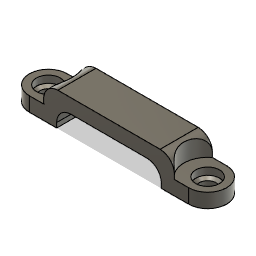
wireholder (Autodesk Fusion 360 design; units mm, degrees)
Autodesk Fusion 360 part; units mm, degrees
note: some values were not read from the file. Set by a fixed rule: which sketch regions a step uses.
sketch "Sketch1" plane through (0, 0, 0) normal (0, 1, 0) x (1, 0, 0)
  line L0 (0, 0) -> (33.5, 0)
  circle A0 centre (0, 0) radius 1.75
  circle A1 centre (33.5, 0) radius 1.75
  circle A2 centre (33.5, 0) radius 4
  circle A3 centre (0, 0) radius 4
  line L1 (0, 4) -> (33.5, 4)
  line L2 (33.5, -4) -> (0, -4)
  dimension "d1" = 33.5
  dimension "d2" = 3.5
  dimension "d3" = 3.5
  dimension "d4" = 8
  dimension "d5" = 8
  constraint coincident L0.start A0.centre
  constraint horizontal L0
  constraint coincident L0.end A1.centre
  constraint concentric A1 A2
  constraint coincident A3 L1.start
  constraint coincident A2 L1.end
  constraint tangent A2 L1
  constraint parallel L0 L1
  constraint coincident A2 L2.start
  constraint coincident A3 L2.end
  constraint tangent A3 L2
  constraint parallel L1 L2
  measures "d1" distance of L0.start L0.end
  measures "d2" diameter of A0
  measures "d3" diameter of A1
  measures "d4" diameter of A2
  measures "d5" diameter of A3
extrude "Extrude1" add sketch "Sketch1" along normal blind 3 makes body 1
hole "Hole1" at (0, 3, 0) direction (0, -1, 0) diameter 5 depth 1.5 tip angle 118 bodies 1
hole "Hole2" at (33.5, 3, 0) direction (0, -1, 0) diameter 5 depth 1.5 tip angle 118 bodies 1
sketch "Sketch9" plane through (0, 3, 0) normal (0, 1, 0) x (-1, 0, 0)
  circle A0 centre (-33.5, 0) radius 2.5
  circle A1 centre (0, 0) radius 2.5
  arc A2 (0, -4) -> (0, 4) centre (0, 0) ccw
  line L0 (0, 4) -> (-33.5, 4)
  arc A3 (-33.5, 4) -> (-33.5, -4) centre (-33.5, 0) ccw
  line L1 (-33.5, -4) -> (0, -4)
  line L2 (-16.75, 4) -> (-5.75, 4)
  line L3 (-16.75, 4) -> (-27.75, 4)
  line L4 (-27.75, 4) -> (-27.75, -4)
  line L5 (-5.75, 4) -> (-5.75, -4)
  circle A4 centre (0, 0) radius 5
  circle A5 centre (-33.5, 0) radius 5
  dimension "d79" = 11
  dimension "d80" = 11
  dimension "d81" = 10
  dimension "d82" = 10
  constraint midpoint L0 L2.start
  constraint parallel L0 L2
  constraint parallel L0 L3
  constraint coincident L1 L4.end
  constraint perpendicular L1 L4
  constraint coincident L1 L5.end
  constraint perpendicular L1 L5
  constraint coincident A1.centre A2.centre
  constraint concentric A0 A5
  measures "d79" distance of L2.start L2.end
  measures "d80" distance of L2.start L3.end
  measures "d81" diameter of A4
  measures "d82" diameter of A5
extrude "Extrude13" add sketch "Sketch9" along normal blind 4 contours L0 L1 L5 A4 | L0 L1 L4 A5 bodies 1
extrude "Extrude14" cut sketch "Sketch9" against normal blind 3 contours L0 L1 L2 L3 L4 L5 bodies 1 makes body 2 at (4.4167, 0, 0)
sketch "Sketch10" plane through (5.75, 0, 0) normal (1, 0, 0) x (0, 0, -1)
  line L0 (4, 0) -> (4, 7)
  line L1 (4, 7) -> (-4, 7)
  line L2 (-4, 7) -> (-4, 0)
  line L3 (-4, 0) -> (4, 0)
  line L4 (-4, 7) -> (4, 7)
  line L5 (4, 7) -> (4, 4)
  line L6 (4, 4) -> (-4, 4)
  line L7 (-4, 4) -> (-4, 7)
  dimension "d87" = 3
  constraint horizontal L4
  constraint vertical L5
  constraint horizontal L6
  constraint vertical L7
  constraint coincident L1.end L2.start
  measures "d87" distance of L1.end L6.end
extrude "Extrude15" add sketch "Sketch10" along normal blind 22 contours L0 L1 L2 L4 L5 L6 L7 bodies 1 2
sketch "Sketch11" plane through (0, 0, 4) normal (0, 0, 1) x (1, 0, 0)
  line L0 (30.5, 7) -> (3, 7)
  line L1 (3, 7) -> (3, 3)
  line L2 (33.5, 3) -> (30.5, 3)
  line L3 (0, 3) -> (0, 0)
  line L4 (27.75, 0) -> (33.5, 0)
  line L5 (5.75, 0) -> (5.75, 4)
  line L6 (5.75, 4) -> (27.75, 4)
  line L7 (5.75, 4) -> (3, 4)
  line L8 (3, 4) -> (6, 4)
  arc A0 (6, 7) -> (3, 4) centre (6, 4) ccw
  line L9 (27.75, 4) -> (27.75, 0)
  line L10 (33.5, 0) -> (33.5, 3)
  line L11 (30.5, 3) -> (30.5, 7)
  line L12 (3, 3) -> (0, 3)
  line L13 (0, 0) -> (5.75, 0)
  line L14 (30.5, 4) -> (27.5, 4)
  arc A1 (30.5, 4) -> (27.5, 7) centre (27.5, 4) ccw
  dimension "d90" = 3
  dimension "d101" = 3
  constraint coincident L5.end L6.start
  constraint coincident L1 L7.end
  constraint perpendicular L1 L7
  constraint perpendicular L1 L8
  constraint coincident L8.end A0.centre
  constraint coincident L11 L14.start
  constraint perpendicular L11 L14
  constraint coincident L0 A1.end
  constraint coincident L14.end A1.centre
  measures "d90" distance of L7.end L8.end
  measures "d101" distance of L14.start L14.end
extrude "Extrude16" cut sketch "Sketch11" against normal blind 10 contours L0 L11 A1 | L0 L1 A0 bodies 1
sketch "Sketch12" plane through (0, 0, 4) normal (0, 0, 1) x (1, 0, 0)
  line L0 (27.75, 4) -> (27.75, 0)
  line L1 (0, 0) -> (5.75, 0)
  line L2 (33.5, 0) -> (33.5, 3)
  line L3 (3, 3) -> (0, 3)
  line L4 (30.5, 3) -> (30.5, 4)
  line L5 (27.5, 7) -> (6, 7)
  line L6 (27.75, 4) -> (24.75, 4)
  line L7 (24.75, 4) -> (24.75, 1)
  arc A0 (27.75, 1) -> (24.75, 4) centre (24.75, 1) ccw
  arc A1 (6, 7) -> (3, 4) centre (6, 4) ccw
  line L8 (3, 4) -> (3, 3)
  line L9 (0, 3) -> (0, 0)
  line L10 (5.75, 0) -> (5.75, 4)
  line L11 (5.75, 4) -> (27.75, 4)
  arc A2 (30.5, 4) -> (27.5, 7) centre (27.5, 4) ccw
  line L12 (27.75, 0) -> (33.5, 0)
  line L13 (33.5, 3) -> (30.5, 3)
  line L14 (5.75, 4) -> (8.75, 4)
  line L15 (8.75, 4) -> (8.75, 1)
  arc A3 (8.75, 4) -> (5.75, 1) centre (8.75, 1) ccw
  dimension "d94" = 3
  dimension "d95" = 3
  dimension "d102" = 3
  dimension "d103" = 3
  constraint coincident L0.start L6.start
  constraint perpendicular L0 L6
  constraint perpendicular L6 L7
  constraint coincident L7.end A0.centre
  constraint coincident L10.end L11.start
  constraint perpendicular L10 L14
  constraint perpendicular L11 L15
  constraint coincident L10 A3.end
  constraint coincident L15.end A3.centre
  measures "d94" distance of L0.start L6.end
  measures "d95" distance of L6.end L7.end
  measures "d102" distance of L10.end L14.end
  measures "d103" distance of L14.end L15.end
extrude "Extrude17" add sketch "Sketch12" against normal blind 8 contours L0 L6 A0 L11 | L10 L11 L14 A3 bodies 1
